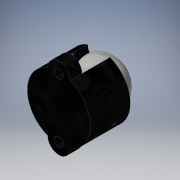
# Autodesk Inventor part: Mini-Q Ball caster
Saved by Autodesk Inventor 2019 (Build 230136000, 136)
## iProperties
Created: 2021-01-09
Part Number: Mini-Q Ball caster
Material: ABS Plastic
Document SubType Name: Modeling
Designer: Sam
Density: 1.06 g/cm^3
Appearance: Smooth - White
Author: Sam
Autodesk Inventor part; units mm, degrees
ref_plane "YZ Plane" through (0, 0, 0) normal (1, 0, 0) x (0, 1, 0)
ref_plane "XZ Plane" through (0, 0, 0) normal (0, 1, 0) x (-1, 0, 0)
ref_plane "XY Plane" through (0, 0, 0) normal (0, 0, 1) x (1, 0, 0)
sketch "Sketch1" plane through (0, 0, 0) normal (0, 0, 1) x (1, 0, 0)
  circle A0 centre (0, 0) radius 7.875
  line L0 (0, 0) -> (8.72, 0)
  circle A1 centre (0, 7.366) radius 2.795
  circle A2 centre (0, -7.366) radius 2.795
  dimension "d0" = 14.732
  dimension "d1" = 15.75
  dimension "d2" = 5.59
  constraints: 3 centre point, 3 coincident, 2 end point, 1 equal radius, 1 horizontal, 1 symmetric about line, 1 vertical alignment
  measures "d0" distance of point (0, -7.366) point (0, 7.366)
  measures "d1" diameter of A0
  measures "d2" diameter of A2
extrude "Extrusion1" add sketch "Sketch1" against normal blind 10
sketch "Sketch2" plane through (0, 0, -10) normal (0, 0, -1) x (-1, 0, 0)
  arc A0 (-2.795, -7.3623) -> (2.795, -7.3623) centre (0, -7.366) ccw projected
  arc A1 (2.795, 7.3623) -> (-2.795, 7.3623) centre (0, 7.366) ccw projected
  circle A2 centre (0, -7.366) radius 2.795
  arc A3 (2.795, -7.3623) -> (2.795, 7.3623) centre (0, 0) ccw projected
  circle A4 centre (0, 7.366) radius 2.795
  constraints: 2 coincident, 1 centre point, 1 concentric, 3 other
extrude "Extrusion2" cut sketch "Sketch2" against normal blind 7
sketch "Sketch3" plane through (0, 0, -3) normal (0, 0, -1) x (-1, 0, 0)
  arc A0 (2.795, 7.3623) -> (-2.795, 7.3623) centre (0, 7.366) ccw projected
  arc A1 (-2.795, -7.3623) -> (2.795, -7.3623) centre (0, -7.366) ccw projected
  point P0 (0, 0)
  constraints: 2 coincident
hole "Hole1" at (0, 7.366, -3) at (0, -7.366, -3) direction (0, 0, 1) diameter 2.3 depth 8 tip angle 118
sketch "Sketch4" plane through (0, 0, 0) normal (1, 0, 0) x (0, 1, 0)
  line L0 (7.3623, 0) -> (7.3623, -3) projected
  line L1 (7.3623, 0) -> (-7.3623, 0) projected
  line L2 (-7.3623, -3) -> (-7.3623, 0) projected
  line L3 (-7.3623, -10) -> (-7.3623, -3) projected
  line L4 (7.3623, -10) -> (-7.3623, -10) projected
  line L5 (7.3623, -3) -> (7.3623, -10) projected
  circle A0 centre (0, -9.24) radius 6.35
  line L6 (0, -9.24) -> (0, -18.9393)
  line L7 (0, -15.59) -> (0, -2.89)
  point P0 (0, 0)
  dimension "d14" = 12.7
  dimension "d15" = 9.24
  constraints: 4 end point, 2 point on circle, 2 point on line, 1 centre point, 1 vertical, 1 vertical alignment
  measures "d14" diameter of A0
  measures "d15" distance of point (0, 0) L6.start
revolve "Revolution1" add sketch "Sketch4" angle 360 about axis through (0, 0, -9.24) along (0, 0, -1) separate body picked at (4.0811, -10.4958) picked at (0.471, -5.0597) contours A0 L6 L4 | L4 L6 L7 A0
body "Solid1"
body "Solid2"
